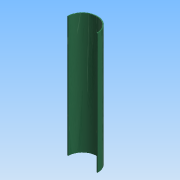
# Autodesk Inventor part: Half Cylinder
Saved by Autodesk Inventor 2018.1 (Build 221171000, 171)
## iProperties
Part Number: Half Cylinder
Material: PMMA Plastic
Document SubType Name: Modeling
Designer: James
Density: 1.188 g/cm^3
Appearance: Smooth - Dark Sea Green
Author: James
Autodesk Inventor part; units mm, degrees
ref_plane "YZ Plane" through (0, 0, 0) normal (1, 0, 0) x (0, 1, 0)
ref_plane "XZ Plane" through (0, 0, 0) normal (0, 1, 0) x (-1, 0, 0)
ref_plane "XY Plane" through (0, 0, 0) normal (0, 0, 1) x (1, 0, 0)
sketch "Sketch1" plane through (0, 0, 0) normal (0, 1, 0) x (-1, 0, 0)
  circle A0 centre (0, 0) radius 250
  circle A1 centre (0, 0) radius 235
  line L0 (235, 0) -> (250, 0)
  line L1 (-235, 0) -> (-250, 0)
  dimension "d0" = 500
  dimension "d1" = 470
  constraints: 4 end point, 4 point on circle, 3 coincident, 2 centre point, 2 point on line, 1 horizontal, 1 horizontal alignment
  measures "d0" diameter of A0
  measures "d1" diameter of A1
extrude "Extrusion1" add sketch "Sketch1" along normal blind 2000 contours A0 L1 A1 L0 picked at (244.6829, -7.263)
body "Solid1"
